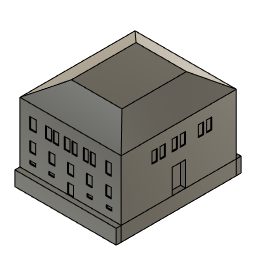
DurantHall v1 (Autodesk Fusion 360 design; units mm, degrees)
Autodesk Fusion 360 part; units mm, degrees
sketch "Sketch1" plane through (0, 0, 0) normal (0, 0, 1) x (1, 0, 0)
  line L0 (1.2905, 0) -> (27.0326, 0)
  line L1 (27.0326, 0) -> (27.0326, 29.2676)
  line L2 (27.0326, 29.2676) -> (1.2905, 29.2676)
  line L3 (1.2905, 29.2676) -> (1.2905, 0)
  constraint horizontal L0
  constraint vertical L1
  constraint horizontal L2
  constraint vertical L3
extrude "Extrude1" add sketch "Sketch1" along normal blind 19.05 makes body 1
ref_plane "WorkPlane1" through (14.1615, 14.6338, 22.86) normal (0, 0, 1) x (1, 0, 0)
sketch "Sketch2" plane through (14.1615, 14.6338, 22.86) normal (0, 0, 1) x (1, 0, 0)
  line L0 (-6.3641, 8.3787) -> (6.4474, 8.3787)
  line L1 (6.4474, 8.3787) -> (6.4474, -8.02)
  line L2 (6.4474, -8.02) -> (-6.3641, -8.02)
  line L3 (-6.3641, -8.02) -> (-6.3641, 8.3787)
  constraint horizontal L0
  constraint vertical L1
  constraint horizontal L2
  constraint vertical L3
loft "Loft1" add profiles "Sketch2" section 1 face at (9.8712, 19.5118, 19.05) section 2 on bodies 1 bodies 1
sketch "Sketch3" plane through (0, 0, 0) normal (0, -1, 0) x (1, 0, 0)
  line L0 (1.2905, 0) -> (27.0326, 0)
  line L1 (27.0326, 0) -> (27.0326, 19.05)
  line L2 (27.0326, 19.05) -> (1.2905, 19.05)
  line L3 (1.2905, 19.05) -> (1.2905, 0)
  line L4 (3.7441, 16.089) -> (5.4317, 16.089)
  line L5 (5.4317, 16.089) -> (5.4317, 13.2394)
  line L6 (5.4317, 13.2394) -> (3.7441, 13.2394)
  line L7 (3.7441, 13.2394) -> (3.7441, 16.089)
  line L8 (7.7834, 16.089) -> (9.3327, 16.089)
  line L9 (9.3327, 16.089) -> (9.3327, 13.2394)
  line L10 (9.3327, 13.2394) -> (7.7834, 13.2394)
  line L11 (7.7834, 13.2394) -> (7.7834, 16.089)
  line L12 (9.7477, 16.089) -> (11.131, 16.089)
  line L13 (11.131, 16.089) -> (11.131, 13.2394)
  line L14 (11.131, 13.2394) -> (9.7477, 13.2394)
  line L15 (9.7477, 13.2394) -> (9.7477, 16.089)
  line L16 (12.5697, 16.089) -> (14.036, 16.089)
  line L17 (14.036, 16.089) -> (14.036, 13.2394)
  line L18 (14.036, 13.2394) -> (12.5697, 13.2394)
  line L19 (12.5697, 13.2394) -> (12.5697, 16.089)
  line L20 (14.534, 16.089) -> (15.8067, 16.089)
  line L21 (15.8067, 16.089) -> (15.8067, 13.2394)
  line L22 (15.8067, 13.2394) -> (14.534, 13.2394)
  line L23 (14.534, 13.2394) -> (14.534, 16.089)
  line L24 (17.4113, 16.089) -> (18.6563, 16.089)
  line L25 (18.6563, 16.089) -> (18.6563, 13.2394)
  line L26 (18.6563, 13.2394) -> (17.4113, 13.2394)
  line L27 (17.4113, 13.2394) -> (17.4113, 16.089)
  line L28 (19.182, 16.089) -> (20.4546, 16.089)
  line L29 (20.4546, 16.089) -> (20.4546, 13.2394)
  line L30 (20.4546, 13.2394) -> (19.182, 13.2394)
  line L31 (19.182, 13.2394) -> (19.182, 16.089)
  line L32 (23.1106, 16.089) -> (24.5216, 16.089)
  line L33 (24.5216, 16.089) -> (24.5216, 13.2394)
  line L34 (24.5216, 13.2394) -> (23.1106, 13.2394)
  line L35 (23.1106, 13.2394) -> (23.1106, 16.089)
  line L36 (23.1106, 10.8047) -> (24.5216, 10.8047)
  line L37 (24.5216, 10.8047) -> (24.5216, 8.287)
  line L38 (24.5216, 8.287) -> (23.1106, 8.287)
  line L39 (23.1106, 8.287) -> (23.1106, 10.8047)
  line L40 (18.186, 10.8047) -> (19.6523, 10.8047)
  line L41 (19.6523, 10.8047) -> (19.6523, 8.287)
  line L42 (19.6523, 8.287) -> (18.186, 8.287)
  line L43 (18.186, 8.287) -> (18.186, 10.8047)
  line L44 (13.3997, 10.8047) -> (14.949, 10.8047)
  line L45 (14.949, 10.8047) -> (14.949, 8.287)
  line L46 (14.949, 8.287) -> (13.3997, 8.287)
  line L47 (13.3997, 8.287) -> (13.3997, 10.8047)
  line L48 (8.641, 10.8047) -> (10.1627, 10.8047)
  line L49 (10.1627, 10.8047) -> (10.1627, 8.287)
  line L50 (10.1627, 8.287) -> (8.641, 8.287)
  line L51 (8.641, 8.287) -> (8.641, 10.8047)
  line L52 (3.7994, 10.8047) -> (5.2934, 10.8047)
  line L53 (5.2934, 10.8047) -> (5.2934, 8.287)
  line L54 (5.2934, 8.287) -> (3.7994, 8.287)
  line L55 (3.7994, 8.287) -> (3.7994, 10.8047)
  line L56 (3.7994, 6.4057) -> (5.2934, 6.4057)
  line L57 (5.2934, 6.4057) -> (5.2934, 5.6587)
  line L58 (5.2934, 5.6587) -> (3.7994, 5.6587)
  line L59 (3.7994, 5.6587) -> (3.7994, 6.4057)
  line L60 (8.6134, 6.4057) -> (9.9967, 6.4057)
  line L61 (9.9967, 6.4057) -> (9.9967, 5.6587)
  line L62 (9.9967, 5.6587) -> (8.6134, 5.6587)
  line L63 (8.6134, 5.6587) -> (8.6134, 6.4057)
  line L64 (13.4273, 6.4057) -> (14.9213, 6.4057)
  line L65 (14.9213, 6.4057) -> (14.9213, 3.7221)
  line L66 (14.9213, 3.7221) -> (13.4273, 3.7221)
  line L67 (13.4273, 3.7221) -> (13.4273, 6.4057)
  line L68 (18.352, 6.4057) -> (19.68, 6.4057)
  line L69 (19.68, 6.4057) -> (19.68, 5.6587)
  line L70 (19.68, 5.6587) -> (18.352, 5.6587)
  line L71 (18.352, 5.6587) -> (18.352, 6.4057)
  line L72 (23.249, 6.4057) -> (24.6323, 6.4057)
  line L73 (24.6323, 6.4057) -> (24.6323, 5.6587)
  line L74 (24.6323, 5.6587) -> (23.249, 5.6587)
  line L75 (23.249, 5.6587) -> (23.249, 6.4057)
  constraint horizontal L4
  constraint vertical L5
  constraint horizontal L6
  constraint vertical L7
  constraint horizontal L8
  constraint vertical L9
  constraint horizontal L10
  constraint vertical L11
  constraint horizontal L12
  constraint vertical L13
  constraint horizontal L14
  constraint vertical L15
  constraint horizontal L16
  constraint vertical L17
  constraint horizontal L18
  constraint vertical L19
  constraint horizontal L20
  constraint vertical L21
  constraint horizontal L22
  constraint vertical L23
  constraint horizontal L24
  constraint vertical L25
  constraint horizontal L26
  constraint vertical L27
  constraint horizontal L28
  constraint vertical L29
  constraint horizontal L30
  constraint vertical L31
  constraint horizontal L32
  constraint vertical L33
  constraint horizontal L34
  constraint vertical L35
  constraint horizontal L36
  constraint vertical L37
  constraint horizontal L38
  constraint vertical L39
  constraint horizontal L40
  constraint vertical L41
  constraint horizontal L42
  constraint vertical L43
  constraint horizontal L44
  constraint vertical L45
  constraint horizontal L46
  constraint vertical L47
  constraint horizontal L48
  constraint vertical L49
  constraint horizontal L50
  constraint vertical L51
  constraint horizontal L52
  constraint vertical L53
  constraint horizontal L54
  constraint vertical L55
  constraint horizontal L56
  constraint vertical L57
  constraint horizontal L58
  constraint vertical L59
  constraint horizontal L60
  constraint vertical L61
  constraint horizontal L62
  constraint vertical L63
  constraint horizontal L64
  constraint vertical L65
  constraint horizontal L66
  constraint vertical L67
  constraint horizontal L68
  constraint vertical L69
  constraint horizontal L70
  constraint vertical L71
  constraint horizontal L72
  constraint vertical L73
  constraint horizontal L74
  constraint vertical L75
extrude "Extrude2" cut sketch "Sketch3" against normal blind 0.254 contours L4 L5 L6 L7 | L8 L9 L10 L11 | L12 L13 L14 L15 | L16 L17 L18 L19 | L20 L21 L22 L23 | L24 L25 L26 L27 | L28 L29 L30 L31 | L32 L33 L34 L35 | L36 L37 L38 L39 | L40 L41 L42 L43 | L44 L45 L46 L47 | L48 L49 L50 L51 | L52 L53 L54 L55 | L56 L57 L58 L59 | L60 L61 L62 L63 | L64 L65 L66 L67 | L68 L69 L70 L71 | L72 L73 L74 L75 bodies 1
sketch "Sketch4" plane through (0, 0, 0) normal (0, -1, 0) x (1, 0, 0)
  line L0 (15.8067, 16.089) -> (15.8067, 13.2394)
  line L1 (15.8067, 13.2394) -> (14.534, 13.2394)
  line L2 (14.534, 13.2394) -> (14.534, 16.089)
  line L3 (14.534, 16.089) -> (15.8067, 16.089)
  line L4 (5.4317, 16.089) -> (5.4317, 13.2394)
  line L5 (5.4317, 13.2394) -> (3.7441, 13.2394)
  line L6 (3.7441, 13.2394) -> (3.7441, 16.089)
  line L7 (3.7441, 16.089) -> (5.4317, 16.089)
  line L8 (9.9967, 6.4057) -> (9.9967, 5.6587)
  line L9 (9.9967, 5.6587) -> (8.6134, 5.6587)
  line L10 (8.6134, 5.6587) -> (8.6134, 6.4057)
  line L11 (8.6134, 6.4057) -> (9.9967, 6.4057)
  line L12 (19.68, 6.4057) -> (19.68, 5.6587)
  line L13 (19.68, 5.6587) -> (18.352, 5.6587)
  line L14 (18.352, 5.6587) -> (18.352, 6.4057)
  line L15 (18.352, 6.4057) -> (19.68, 6.4057)
  line L16 (24.5216, 16.089) -> (24.5216, 13.2394)
  line L17 (24.5216, 13.2394) -> (23.1106, 13.2394)
  line L18 (23.1106, 13.2394) -> (23.1106, 16.089)
  line L19 (23.1106, 16.089) -> (24.5216, 16.089)
  line L20 (19.6523, 10.8047) -> (19.6523, 8.287)
  line L21 (19.6523, 8.287) -> (18.186, 8.287)
  line L22 (18.186, 8.287) -> (18.186, 10.8047)
  line L23 (18.186, 10.8047) -> (19.6523, 10.8047)
  line L24 (5.2934, 6.4057) -> (5.2934, 5.6587)
  line L25 (5.2934, 5.6587) -> (3.7994, 5.6587)
  line L26 (3.7994, 5.6587) -> (3.7994, 6.4057)
  line L27 (3.7994, 6.4057) -> (5.2934, 6.4057)
  line L28 (9.3327, 16.089) -> (9.3327, 13.2394)
  line L29 (9.3327, 13.2394) -> (7.7834, 13.2394)
  line L30 (7.7834, 13.2394) -> (7.7834, 16.089)
  line L31 (7.7834, 16.089) -> (9.3327, 16.089)
  line L32 (18.6563, 16.089) -> (18.6563, 13.2394)
  line L33 (18.6563, 13.2394) -> (17.4113, 13.2394)
  line L34 (17.4113, 13.2394) -> (17.4113, 16.089)
  line L35 (17.4113, 16.089) -> (18.6563, 16.089)
  line L36 (14.036, 16.089) -> (14.036, 13.2394)
  line L37 (14.036, 13.2394) -> (12.5697, 13.2394)
  line L38 (12.5697, 13.2394) -> (12.5697, 16.089)
  line L39 (12.5697, 16.089) -> (14.036, 16.089)
  line L40 (10.1627, 10.8047) -> (10.1627, 8.287)
  line L41 (10.1627, 8.287) -> (8.641, 8.287)
  line L42 (8.641, 8.287) -> (8.641, 10.8047)
  line L43 (8.641, 10.8047) -> (10.1627, 10.8047)
  line L44 (14.9213, 6.4057) -> (14.9213, 3.7221)
  line L45 (14.9213, 3.7221) -> (13.4273, 3.7221)
  line L46 (13.4273, 3.7221) -> (13.4273, 6.4057)
  line L47 (13.4273, 6.4057) -> (14.9213, 6.4057)
  line L48 (24.6323, 6.4057) -> (24.6323, 5.6587)
  line L49 (24.6323, 5.6587) -> (23.249, 5.6587)
  line L50 (23.249, 5.6587) -> (23.249, 6.4057)
  line L51 (23.249, 6.4057) -> (24.6323, 6.4057)
  line L52 (24.5216, 10.8047) -> (24.5216, 8.287)
  line L53 (24.5216, 8.287) -> (23.1106, 8.287)
  line L54 (23.1106, 8.287) -> (23.1106, 10.8047)
  line L55 (23.1106, 10.8047) -> (24.5216, 10.8047)
  line L56 (14.949, 10.8047) -> (14.949, 8.287)
  line L57 (14.949, 8.287) -> (13.3997, 8.287)
  line L58 (13.3997, 8.287) -> (13.3997, 10.8047)
  line L59 (13.3997, 10.8047) -> (14.949, 10.8047)
  line L60 (5.2934, 10.8047) -> (5.2934, 8.287)
  line L61 (5.2934, 8.287) -> (3.7994, 8.287)
  line L62 (3.7994, 8.287) -> (3.7994, 10.8047)
  line L63 (3.7994, 10.8047) -> (5.2934, 10.8047)
  line L64 (11.131, 16.089) -> (11.131, 13.2394)
  line L65 (11.131, 13.2394) -> (9.7477, 13.2394)
  line L66 (9.7477, 13.2394) -> (9.7477, 16.089)
  line L67 (9.7477, 16.089) -> (11.131, 16.089)
  line L68 (20.4546, 16.089) -> (20.4546, 13.2394)
  line L69 (20.4546, 13.2394) -> (19.182, 13.2394)
  line L70 (19.182, 13.2394) -> (19.182, 16.089)
  line L71 (19.182, 16.089) -> (20.4546, 16.089)
  line L72 (1.2905, 0) -> (27.0326, 0)
  line L73 (27.0326, 0) -> (27.0326, 19.05)
  line L74 (27.0326, 19.05) -> (1.2905, 19.05)
  line L75 (1.2905, 19.05) -> (1.2905, 0)
  line L76 (-0.8297, 3.7221) -> (28.3392, 3.7221)
  line L77 (28.3392, 3.7221) -> (28.3392, 0.0038)
  line L78 (28.3392, 0.0038) -> (-0.8297, 0.0038)
  line L79 (-0.8297, 0.0038) -> (-0.8297, 3.7221)
  constraint horizontal L76
  constraint vertical L77
  constraint horizontal L78
  constraint vertical L79
extrude "Extrude3" add sketch "Sketch4" against normal blind 30.48 separate body contours L45 L73 L75 L76 L78 makes body 2
extrude "Extrude4" add 1 faces at (13.9168, 30.48, 1.2432) along direction (0, -1, 0) blind 31.75 separate body on bodies 2 makes body 3
sketch "Sketch5" plane through (27.0326, 0, 0) normal (1, 0, 0) x (0, 1, 0)
  line L0 (0, 0) -> (29.2676, 0)
  line L1 (29.2676, 0) -> (29.2676, 19.05)
  line L2 (29.2676, 19.05) -> (0, 19.05)
  line L3 (0, 19.05) -> (0, 0)
  line L4 (14.2857, 16.2228) -> (12.969, 16.2228)
  line L5 (12.969, 16.2228) -> (12.969, 13.3758)
  line L6 (12.969, 13.3758) -> (14.2857, 13.3758)
  line L7 (14.2857, 13.3758) -> (14.2857, 16.2228)
  line L8 (15.0399, 16.2228) -> (16.3607, 16.2228)
  line L9 (16.3607, 16.2228) -> (16.3607, 13.3758)
  line L10 (16.3607, 13.3758) -> (15.0399, 13.3758)
  line L11 (15.0399, 13.3758) -> (15.0399, 16.2228)
  line L12 (9.1619, 13.2554) -> (9.1619, 16.1024)
  line L13 (11.2369, 16.1024) -> (11.2369, 13.2554)
  line L14 (9.9161, 13.2554) -> (9.9161, 16.1024)
  line L15 (9.1619, 16.1024) -> (7.8452, 16.1024)
  line L16 (7.8452, 16.1024) -> (7.8452, 13.2554)
  line L17 (9.9161, 16.1024) -> (11.2369, 16.1024)
  line L18 (11.2369, 13.2554) -> (9.9161, 13.2554)
  line L19 (7.8452, 13.2554) -> (9.1619, 13.2554)
  line L20 (14.2857, 13.3758) -> (14.2857, 16.2228)
  line L21 (16.3607, 16.2228) -> (16.3607, 13.3758)
  line L22 (15.0399, 13.3758) -> (15.0399, 16.2228)
  line L23 (14.2857, 16.2228) -> (12.969, 16.2228)
  line L24 (12.969, 16.2228) -> (12.969, 13.3758)
  line L25 (15.0399, 16.2228) -> (16.3607, 16.2228)
  line L26 (16.3607, 13.3758) -> (15.0399, 13.3758)
  line L27 (12.969, 13.3758) -> (14.2857, 13.3758)
  line L28 (23.0282, 16.0696) -> (23.0282, 13.2225)
  line L29 (20.9532, 13.2225) -> (20.9532, 16.0696)
  line L30 (21.7074, 13.2225) -> (21.7074, 16.0696)
  line L31 (21.7074, 13.2225) -> (21.7074, 16.0696)
  line L32 (21.7074, 16.0696) -> (23.0282, 16.0696)
  line L33 (19.6365, 13.2225) -> (20.9532, 13.2225)
  line L34 (23.0282, 13.2225) -> (21.7074, 13.2225)
  line L35 (20.9532, 16.0696) -> (19.6365, 16.0696)
  line L36 (19.6365, 16.0696) -> (19.6365, 13.2225)
  line L37 (20.9532, 16.0696) -> (19.6365, 16.0696)
  line L38 (23.0282, 13.2225) -> (21.7074, 13.2225)
  line L39 (20.9532, 13.2225) -> (20.9532, 16.0696)
  line L40 (23.0282, 16.0696) -> (23.0282, 13.2225)
  line L41 (19.6365, 13.2225) -> (20.9532, 13.2225)
  line L42 (19.6365, 16.0696) -> (19.6365, 13.2225)
  line L43 (21.7074, 16.0696) -> (23.0282, 16.0696)
  dimension "d11" = 1.3208
  dimension "d12" = 1.3208
  dimension "d13" = 1.3208
  dimension "d14" = 1.3208
  dimension "d15" = 1.3208
  constraint horizontal L4
  constraint vertical L5
  constraint horizontal L6
  constraint vertical L7
  constraint horizontal L8
  constraint vertical L9
  constraint horizontal L10
  constraint vertical L11
  constraint horizontal L15
  constraint vertical L16
  constraint horizontal L19
  constraint vertical L12
  constraint horizontal L17
  constraint vertical L13
  constraint horizontal L18
  constraint vertical L14
  constraint horizontal L23
  constraint vertical L24
  constraint horizontal L27
  constraint vertical L20
  constraint horizontal L25
  constraint vertical L21
  constraint horizontal L26
  constraint vertical L22
  constraint horizontal L35
  constraint vertical L36
  constraint horizontal L41
  constraint vertical L39
  constraint horizontal L32
  constraint vertical L40
  constraint horizontal L38
  constraint vertical L31
  constraint horizontal L37
  constraint vertical L42
  constraint horizontal L33
  constraint vertical L29
  constraint horizontal L43
  constraint vertical L28
  constraint horizontal L34
  constraint vertical L30
  measures "d11" distance of L8.start L8.end
  measures "d12" distance of L14.end L13.start
  measures "d13" distance of L8.start L8.end
  measures "d14" distance of L30.end L28.start
  measures "d15" distance of L30.end L28.start
extrude "Extrude5" cut sketch "Sketch5" against normal blind 0.254 contours L4 L5 L6 L7 L20 L23 L24 L27 | L8 L9 L10 L11 L21 L22 L25 L26 | L12 L15 L16 L19 | L13 L14 L17 L18 | L28 L30 L31 L32 L34 L38 L40 L43 | L29 L33 L35 L36 L37 L39 L41 L42 bodies 1
sketch "Sketch6" plane through (27.0326, 0, 0) normal (1, 0, 0) x (0, 1, 0)
  line L0 (14.2857, 16.2228) -> (14.2857, 13.3758)
  line L1 (14.2857, 13.3758) -> (12.969, 13.3758)
  line L2 (12.969, 13.3758) -> (12.969, 16.2228)
  line L3 (12.969, 16.2228) -> (14.2857, 16.2228)
  line L4 (23.0282, 13.2225) -> (21.7074, 13.2225)
  line L5 (21.7074, 13.2225) -> (21.7074, 16.0696)
  line L6 (21.7074, 16.0696) -> (23.0282, 16.0696)
  line L7 (23.0282, 16.0696) -> (23.0282, 13.2225)
  line L8 (9.9161, 16.1024) -> (11.2369, 16.1024)
  line L9 (11.2369, 16.1024) -> (11.2369, 13.2554)
  line L10 (11.2369, 13.2554) -> (9.9161, 13.2554)
  line L11 (9.9161, 13.2554) -> (9.9161, 16.1024)
  line L12 (15.0399, 16.2228) -> (16.3607, 16.2228)
  line L13 (16.3607, 16.2228) -> (16.3607, 13.3758)
  line L14 (16.3607, 13.3758) -> (15.0399, 13.3758)
  line L15 (15.0399, 13.3758) -> (15.0399, 16.2228)
  line L16 (20.9532, 13.2225) -> (19.6365, 13.2225)
  line L17 (19.6365, 13.2225) -> (19.6365, 16.0696)
  line L18 (19.6365, 16.0696) -> (20.9532, 16.0696)
  line L19 (20.9532, 16.0696) -> (20.9532, 13.2225)
  line L20 (9.1619, 16.1024) -> (9.1619, 13.2554)
  line L21 (9.1619, 13.2554) -> (7.8452, 13.2554)
  line L22 (7.8452, 13.2554) -> (7.8452, 16.1024)
  line L23 (7.8452, 16.1024) -> (9.1619, 16.1024)
  line L24 (0, 0) -> (29.2676, 0)
  line L25 (29.2676, 0) -> (29.2676, 19.05)
  line L26 (29.2676, 19.05) -> (0, 19.05)
  line L27 (0, 19.05) -> (0, 0)
  line L28 (12.969, 3.7488) -> (16.3607, 3.7488)
  line L29 (16.3607, 3.7488) -> (16.3607, 10.031)
  line L30 (16.3607, 10.031) -> (12.969, 10.031)
  line L31 (12.969, 10.031) -> (12.969, 3.7488)
  constraint horizontal L28
  constraint vertical L29
  constraint horizontal L30
  constraint vertical L31
extrude "Extrude6" cut sketch "Sketch6" against normal blind 1.27 contours L28 L29 L30 L31 bodies 1
sketch "Sketch8" plane through (0, 29.2676, 0) normal (0, 1, 0) x (-1, 0, 0)
  line L0 (-27.0326, 0) -> (-1.2905, 0)
  line L1 (-1.2905, 0) -> (-1.2905, 19.05)
  line L2 (-1.2905, 19.05) -> (-27.0326, 19.05)
  line L3 (-27.0326, 19.05) -> (-27.0326, 0)
  line L4 (-24.5276, 16.1089) -> (-23.0443, 16.1089)
  line L5 (-23.0443, 16.1089) -> (-23.0443, 13.2178)
  line L6 (-23.0443, 13.2178) -> (-24.5276, 13.2178)
  line L7 (-24.5276, 13.2178) -> (-24.5276, 16.1089)
  line L8 (-20.4548, 13.2178) -> (-19.1726, 13.2178)
  line L9 (-19.1726, 13.2178) -> (-19.1726, 16.1089)
  line L10 (-19.1726, 16.1089) -> (-20.4548, 16.1089)
  line L11 (-20.4548, 16.1089) -> (-20.4548, 13.2178)
  line L12 (-18.6698, 16.1089) -> (-17.3876, 16.1089)
  line L13 (-17.3876, 16.1089) -> (-17.3876, 13.2178)
  line L14 (-17.3876, 13.2178) -> (-18.6698, 13.2178)
  line L15 (-18.6698, 13.2178) -> (-18.6698, 16.1089)
  line L16 (-15.7786, 13.2178) -> (-14.4713, 13.2178)
  line L17 (-14.4713, 13.2178) -> (-14.4713, 16.1089)
  line L18 (-14.4713, 16.1089) -> (-15.7786, 16.1089)
  line L19 (-15.7786, 16.1089) -> (-15.7786, 13.2178)
  line L20 (-13.9684, 16.1089) -> (-12.5857, 16.1089)
  line L21 (-12.5857, 16.1089) -> (-12.5857, 13.2178)
  line L22 (-12.5857, 13.2178) -> (-13.9684, 13.2178)
  line L23 (-13.9684, 13.2178) -> (-13.9684, 16.1089)
  line L24 (-11.1527, 16.1089) -> (-9.7196, 16.1089)
  line L25 (-9.7196, 16.1089) -> (-9.7196, 13.2178)
  line L26 (-9.7196, 13.2178) -> (-11.1527, 13.2178)
  line L27 (-11.1527, 13.2178) -> (-11.1527, 16.1089)
  line L28 (-9.3174, 13.2178) -> (-7.7587, 13.2178)
  line L29 (-7.7587, 13.2178) -> (-7.7587, 16.1089)
  line L30 (-7.7587, 16.1089) -> (-9.3174, 16.1089)
  line L31 (-9.3174, 16.1089) -> (-9.3174, 13.2178)
  line L32 (-5.3703, 16.1089) -> (-3.7613, 16.1089)
  line L33 (-3.7613, 16.1089) -> (-3.7613, 13.2178)
  line L34 (-3.7613, 13.2178) -> (-5.3703, 13.2178)
  line L35 (-5.3703, 13.2178) -> (-5.3703, 16.1089)
  line L36 (-3.7613, 10.7539) -> (-5.3703, 10.7539)
  line L37 (-5.3703, 10.7539) -> (-5.3703, 8.3404)
  line L38 (-5.3703, 8.3404) -> (-3.7613, 8.3404)
  line L39 (-3.7613, 8.3404) -> (-3.7613, 10.7539)
  line L40 (-8.7391, 8.3404) -> (-10.147, 8.3404)
  line L41 (-10.147, 8.3404) -> (-10.147, 10.7539)
  line L42 (-10.147, 10.7539) -> (-8.7391, 10.7539)
  line L43 (-8.7391, 10.7539) -> (-8.7391, 8.3404)
  line L44 (-13.4405, 10.7539) -> (-14.9741, 10.7539)
  line L45 (-14.9741, 10.7539) -> (-14.9741, 8.3404)
  line L46 (-14.9741, 8.3404) -> (-13.4405, 8.3404)
  line L47 (-13.4405, 8.3404) -> (-13.4405, 10.7539)
  line L48 (-18.167, 8.3404) -> (-19.6754, 8.3404)
  line L49 (-19.6754, 8.3404) -> (-19.6754, 10.7539)
  line L50 (-19.6754, 10.7539) -> (-18.167, 10.7539)
  line L51 (-18.167, 10.7539) -> (-18.167, 8.3404)
  line L52 (-23.1197, 10.7539) -> (-24.5276, 10.7539)
  line L53 (-24.5276, 10.7539) -> (-24.5276, 8.3404)
  line L54 (-24.5276, 8.3404) -> (-23.1197, 8.3404)
  line L55 (-23.1197, 8.3404) -> (-23.1197, 10.7539)
  line L56 (-24.6383, 6.398) -> (-23.2554, 6.398)
  line L57 (-23.2554, 6.398) -> (-23.2554, 5.6284)
  line L58 (-23.2554, 5.6284) -> (-24.6383, 5.6284)
  line L59 (-24.6383, 5.6284) -> (-24.6383, 6.398)
  line L60 (-19.6754, 5.6284) -> (-18.3613, 5.6284)
  line L61 (-18.3613, 5.6284) -> (-18.3613, 6.398)
  line L62 (-18.3613, 6.398) -> (-19.6754, 6.398)
  line L63 (-19.6754, 6.398) -> (-19.6754, 5.6284)
  line L64 (-14.9222, 6.398) -> (-13.4191, 6.398)
  line L65 (-13.4191, 6.398) -> (-13.4191, 3.7284)
  line L66 (-13.4191, 3.7284) -> (-14.9222, 3.7284)
  line L67 (-14.9222, 3.7284) -> (-14.9222, 6.398)
  line L68 (-10.0161, 6.398) -> (-8.6212, 6.398)
  line L69 (-8.6212, 6.398) -> (-8.6212, 5.6284)
  line L70 (-8.6212, 5.6284) -> (-10.0161, 5.6284)
  line L71 (-10.0161, 5.6284) -> (-10.0161, 6.398)
  line L72 (-5.3024, 6.398) -> (-3.7993, 6.398)
  line L73 (-3.7993, 6.398) -> (-3.7993, 5.6284)
  line L74 (-3.7993, 5.6284) -> (-5.3024, 5.6284)
  line L75 (-5.3024, 5.6284) -> (-5.3024, 6.398)
  constraint horizontal L4
  constraint vertical L5
  constraint horizontal L6
  constraint vertical L7
  constraint horizontal L8
  constraint vertical L9
  constraint horizontal L10
  constraint vertical L11
  constraint horizontal L12
  constraint vertical L13
  constraint horizontal L14
  constraint vertical L15
  constraint horizontal L16
  constraint vertical L17
  constraint horizontal L18
  constraint vertical L19
  constraint horizontal L20
  constraint vertical L21
  constraint horizontal L22
  constraint vertical L23
  constraint horizontal L24
  constraint vertical L25
  constraint horizontal L26
  constraint vertical L27
  constraint horizontal L28
  constraint vertical L29
  constraint horizontal L30
  constraint vertical L31
  constraint horizontal L32
  constraint vertical L33
  constraint horizontal L34
  constraint vertical L35
  constraint horizontal L36
  constraint vertical L37
  constraint horizontal L38
  constraint vertical L39
  constraint horizontal L40
  constraint vertical L41
  constraint horizontal L42
  constraint vertical L43
  constraint horizontal L44
  constraint vertical L45
  constraint horizontal L46
  constraint vertical L47
  constraint horizontal L48
  constraint vertical L49
  constraint horizontal L50
  constraint vertical L51
  constraint horizontal L52
  constraint vertical L53
  constraint horizontal L54
  constraint vertical L55
  constraint horizontal L56
  constraint vertical L57
  constraint horizontal L58
  constraint vertical L59
  constraint horizontal L60
  constraint vertical L61
  constraint horizontal L62
  constraint vertical L63
  constraint horizontal L64
  constraint vertical L65
  constraint horizontal L66
  constraint vertical L67
  constraint horizontal L68
  constraint vertical L69
  constraint horizontal L70
  constraint vertical L71
  constraint horizontal L72
  constraint vertical L73
  constraint horizontal L74
  constraint vertical L75
extrude "Extrude7" cut sketch "Sketch8" against normal blind 0.254 contours L4 L5 L6 L7 | L8 L9 L10 L11 | L12 L13 L14 L15 | L16 L17 L18 L19 | L20 L21 L22 L23 | L24 L25 L26 L27 | L28 L29 L30 L31 | L32 L33 L34 L35 | L36 L37 L38 L39 | L40 L41 L42 L43 | L44 L45 L46 L47 | L48 L49 L50 L51 | L52 L53 L54 L55 | L56 L57 L58 L59 | L60 L61 L62 L63 | L64 L65 L66 L67 | L68 L69 L70 L71 | L72 L73 L74 L75 bodies 1
sketch "Sketch9" plane through (1.2905, 0, 0) normal (-1, 0, 0) x (0, -1, 0)
  line L0 (-29.2676, 0) -> (0, 0)
  line L1 (0, 0) -> (0, 19.05)
  line L2 (0, 19.05) -> (-29.2676, 19.05)
  line L3 (-29.2676, 19.05) -> (-29.2676, 0)
  line L4 (-23.0511, 16.065) -> (-21.702, 16.065)
  line L5 (-21.702, 16.065) -> (-21.702, 13.2079)
  line L6 (-21.702, 13.2079) -> (-23.0511, 13.2079)
  line L7 (-23.0511, 13.2079) -> (-23.0511, 16.065)
  line L8 (-20.9678, 16.065) -> (-19.6385, 16.065)
  line L9 (-19.6385, 16.065) -> (-19.6385, 13.2079)
  line L10 (-19.6385, 13.2079) -> (-20.9678, 13.2079)
  line L11 (-20.9678, 13.2079) -> (-20.9678, 16.065)
  line L12 (-11.226, 16.065) -> (-9.9165, 16.065)
  line L13 (-9.9165, 16.065) -> (-9.9165, 13.2079)
  line L14 (-9.9165, 13.2079) -> (-11.226, 13.2079)
  line L15 (-11.226, 13.2079) -> (-11.226, 16.065)
  line L16 (-9.1625, 16.065) -> (-7.8133, 16.065)
  line L17 (-7.8133, 16.065) -> (-7.8133, 13.2079)
  line L18 (-7.8133, 13.2079) -> (-9.1625, 13.2079)
  line L19 (-9.1625, 13.2079) -> (-9.1625, 16.065)
  line L20 (-16.3846, 16.2436) -> (-15.0552, 16.2436)
  line L21 (-15.0552, 16.2436) -> (-15.0552, 13.4063)
  line L22 (-15.0552, 13.4063) -> (-16.3846, 13.4063)
  line L23 (-16.3846, 13.4063) -> (-16.3846, 16.2436)
  line L24 (-14.2815, 16.2436) -> (-13.0116, 16.2436)
  line L25 (-13.0116, 16.2436) -> (-13.0116, 13.4063)
  line L26 (-13.0116, 13.4063) -> (-14.2815, 13.4063)
  line L27 (-14.2815, 13.4063) -> (-14.2815, 16.2436)
  line L28 (-16.3647, 10.0532) -> (-13.0116, 10.0532)
  line L29 (-13.0116, 10.0532) -> (-13.0116, 3.7636)
  line L30 (-13.0116, 3.7636) -> (-16.3647, 3.7636)
  line L31 (-16.3647, 3.7636) -> (-16.3647, 10.0532)
  constraint horizontal L4
  constraint vertical L5
  constraint horizontal L6
  constraint vertical L7
  constraint horizontal L8
  constraint vertical L9
  constraint horizontal L10
  constraint vertical L11
  constraint horizontal L12
  constraint vertical L13
  constraint horizontal L14
  constraint vertical L15
  constraint horizontal L16
  constraint vertical L17
  constraint horizontal L18
  constraint vertical L19
  constraint horizontal L20
  constraint vertical L21
  constraint horizontal L22
  constraint vertical L23
  constraint horizontal L24
  constraint vertical L25
  constraint horizontal L26
  constraint vertical L27
  constraint horizontal L28
  constraint vertical L29
  constraint horizontal L30
  constraint vertical L31
extrude "Extrude8" cut sketch "Sketch9" against normal blind 0.254 contours L4 L5 L6 L7 | L8 L9 L10 L11 | L12 L13 L14 L15 | L16 L17 L18 L19 | L20 L21 L22 L23 | L24 L25 L26 L27 | L28 L29 L30 L31 bodies 1
extrude "Extrude9" cut 1 faces at (1.5445, 15.247, 7.9567) along direction (1, 0, 0) blind 0.762 on bodies 1 bodies 1
